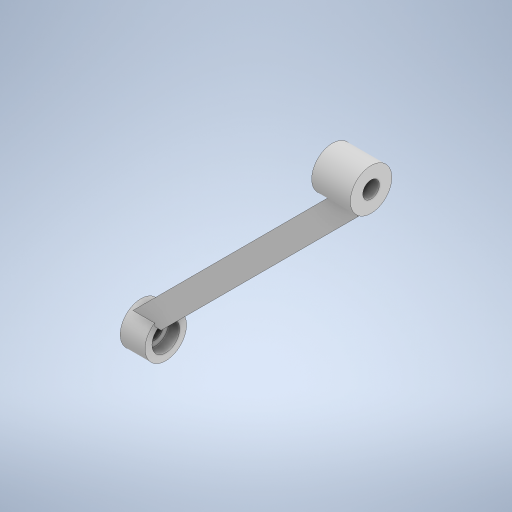
# Autodesk Inventor part: Conector
Saved by Autodesk Inventor 2023 (Build 270158000, 158)
## iProperties
Created: 2022-11-05
Part Number: Conector
Material: Generic
Document SubType Name: Modeling
Designer: ivanm
Density: 1 g/cm^3
Appearance: Default
Author: ivanm
Autodesk Inventor part; units mm, degrees
ref_plane "YZ Plane" through (0, 0, 0) normal (1, 0, 0) x (0, 1, 0)
ref_plane "XZ Plane" through (0, 0, 0) normal (0, 1, 0) x (-1, 0, 0)
sketch "Sketch1" plane through (0, 0, 0) normal (1, 0, 0) x (0, 1, 0)
  circle A0 centre (0, 0) radius 3
  circle A1 centre (0, 0) radius 7.5
  dimension "d0" = 6
  dimension "d1" = 15
  constraints: 2 centre point, 2 coincident
  measures "d0" diameter of A0
  measures "d1" diameter of A1
extrude "Extrusion1" add sketch "Sketch1" along normal blind 14
sketch "Sketch2" plane through (0, 0, 0) normal (0, 0, 1) x (1, 0, 0)
  line L0 (14, -7.5) -> (14, 7.5) projected
  line L1 (0, -7.5) -> (0, 7.5) projected
  line L2 (0, -7.5) -> (14, -7.5) projected
  line L3 (7, -7.5) -> (-63.7107, -78.2107)
  line L4 (13.2599, -6.897) -> (-46.7401, -66.897)
  line L5 (3.7119, -5.1312) -> (-52.397, -61.2401)
  line L6 (-52.397, -61.2401) -> (-58.0538, -66.897)
  line L7 (-63.7107, -78.2107) -> (-58.0538, -78.2107)
  line L8 (-63.7107, -78.2107) -> (-69.3675, -78.2107)
  line L9 (-58.0538, -78.2107) -> (-46.7401, -66.897)
  line L10 (-58.0538, -66.897) -> (-69.3675, -78.2107)
  line L11 (3.7119, -5.1312) -> (12.583, -5.1312)
  line L12 (13.2599, -6.897) -> (12.583, -5.1312)
  point P0 (0, 0)
  point P1 (-58.0538, -78.2107)
  point P2 (1.3431, -7.5)
  point P3 (12.6569, -7.5)
  dimension "d4" = 100
  dimension "d5" = 45
  dimension "d6" = 4
  dimension "d7" = 4
  dimension "d10" = 8.871
  dimension "d12" = 60
  constraints: 20 end point, 4 parallel, 3 horizontal, 1 collinear, 1 midpoint, 1 point on line
  measures "d4" distance of L3.start L3.end
  measures "d5" angle of L2 L3
  measures "d6" distance between parallel lines of L3 L4
  measures "d7" distance between parallel lines of L3 L5
  measures "d10" distance of L5.start L11.end
  measures "d12" horizontal distance of L4.start L4.end
extrude "Extrusion2" add sketch "Sketch2" along normal mid plane 8
extrude "Extrusion3" add sketch "Sketch1" along normal blind 2 contours A0
ref_plane "Work Plane1" through (-69.3675, -78.2107, 0) normal (-1, 0, 0) x (0, 0, 1)
sketch "Sketch3" plane through (-69.3675, -78.2107, 0) normal (-1, 0, 0) x (0, 0, 1)
  arc A0 (-4, 71.8664) -> (4, 71.8664) centre (0, 78.2107) ccw projected
  line L0 (-4, 0) -> (-4, 71.8664) projected
  line L1 (-4, 0) -> (4, 0) projected
  line L2 (4, 71.8664) -> (4, 0) projected
  circle A1 centre (0, -5.241) radius 7.5
  circle A2 centre (0, -5.241) radius 3
  line L3 (0, -32.4313) -> (0, 105.401) projected
  point P0 (0, 0)
  dimension "d15" = 15
  dimension "d16" = 6
  dimension "d17" = 5.241
  constraints: 2 centre point, 1 coincident, 1 midpoint, 1 point on line
  measures "d15" diameter of A1
  measures "d16" diameter of A2
  measures "d17" distance of point (0, 0) A1.centre
extrude "Extrusion4" add sketch "Sketch3" against normal blind 9 contours A1 L3 L1 L0 | L0 L1 L3 A2 A1 | A1 L2 L1 L3 | L3 A2 L1 L2 A1
sketch "Sketch4" plane through (-60.3675, -78.2107, 0) normal (1, 0, 0) x (0, 0, -1)
  circle A0 centre (0, -5.241) radius 3 projected
  circle A1 centre (0, -5.241) radius 5
  point P0 (0, 78.2107)
  dimension "d20" = 10
  constraints: 1 centre point, 1 coincident
  measures "d20" diameter of A1
extrude "Extrusion5" cut sketch "Sketch4" along normal blind 9 and the other way blind 4
body "Solid1"
